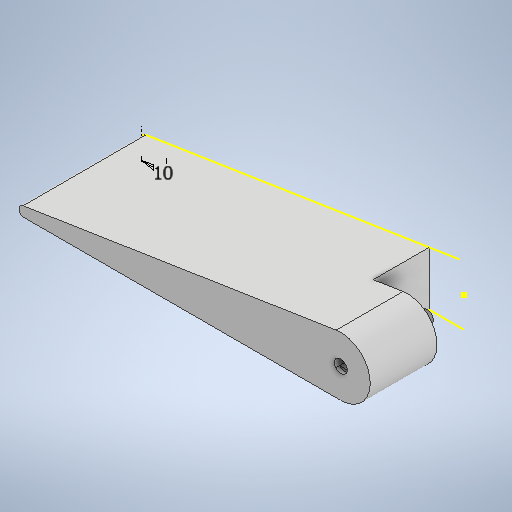
# Autodesk Inventor part: 13042025-02
Saved by Autodesk Inventor 2025.2 (Build 292293000, 293)
## iProperties
Created: 2026-04-13
Part Number: 13042025-02
Material: Generic
Document SubType Name: Modeling
Designer: Oski
Density: 1 g/cm^3
Appearance: Default
Author: Oski
Autodesk Inventor part; units mm, degrees
ref_plane "YZ Plane" through (0, 0, 0) normal (1, 0, 0) x (0, 1, 0)
ref_plane "XZ Plane" through (0, 0, 0) normal (0, 1, 0) x (-1, 0, 0)
ref_plane "XY Plane" through (0, 0, 0) normal (0, 0, 1) x (1, 0, 0)
sketch "Sketch1" plane through (0, 0, 0) normal (0, 0, 1) x (1, 0, 0)
  line L0 (-12, 12) -> (12, 12)
  line L1 (12, 12) -> (12, -12)
  line L2 (12, -12) -> (-12, -12)
  line L3 (-12, -12) -> (-12, 12)
  line L4 (0, 0) -> (0, 12) construction
  line L5 (0, 0) -> (0, -12) construction
  line L6 (0, 0) -> (-12, 0) construction
  dimension "d0" = 24
  dimension "d1" = 24
  constraints: 14 end point, 3 midpoint, 3 perpendicular, 2 equal length, 2 parallel, 1 horizontal, 1 point on line
  measures "d0" distance of L0.start L0.end
  measures "d1" distance of L2.end L0.start
extrude "Extrusion1" add sketch "Sketch1" along normal blind 27.2
fillet "Fillet2" radius 12 4 edges at (12, 12, 13.6) (12, -12, 13.6) (-12, 12, 13.6) (-12, -12, 13.6)
sketch "Sketch2" plane through (0, 0, 27.2) normal (0, 0, 1) x (1, 0, 0)
  line L0 (2.1125, -1.6) -> (-2.1125, -1.6)
  line L1 (2.1125, 1.6) -> (-2.1125, 1.6)
  arc A0 (2.1125, -1.6) -> (2.1125, 1.6) centre (0, 0) ccw
  arc A1 (-2.1125, 1.6) -> (-2.1125, -1.6) centre (0, 0) ccw
  point P0 (2.65, 0)
  point P1 (-2.65, 0)
  dimension "d9" = 2.65
  dimension "d10" = 3.2
  constraints: 6 point on circle, 4 end point, 2 centre point, 2 coincident, 2 horizontal, 1 concentric, 1 parallel
  measures "d9" radius of A0
  measures "d10" distance between parallel lines of L1 L0
extrude "Extrusion2" cut sketch "Sketch2" against normal blind 8
sketch "Sketch3" plane through (0, 0, 27.2) normal (0, 0, 1) x (1, 0, 0)
  circle A0 centre (0, 0) radius 2.6
  dimension "d13" = 5.2
  constraints: 1 centre point, 1 coincident
  measures "d13" diameter of A0
extrude "Extrusion3" cut sketch "Sketch3" against normal blind 1.6
sketch "Sketch4" plane through (0, 0, 0) normal (0, 0, -1) x (-1, 0, 0)
  arc A0 (-2.1125, 1.6) -> (-2.1125, -1.6) centre (0, 0) ccw projected
  circle A1 centre (0, 0) radius 3.25
  dimension "d17" = 6.5
  constraints: 1 centre point, 1 coincident
  measures "d17" diameter of A1
extrude "Extrusion4" add sketch "Sketch4" along normal blind 3
sketch "Sketch5" plane through (0, 0, -3) normal (0, 0, -1) x (-1, 0, 0)
  circle A0 centre (0, 0) radius 2.45
  dimension "d20" = 4.9
  constraints: 1 centre point, 1 coincident
  measures "d20" diameter of A0
extrude "Extrusion5" add sketch "Sketch5" along normal blind 5
sketch "Sketch7" plane through (0, 0, 27.2) normal (0, 0, 1) x (1, 0, 0)
  circle A0 centre (0, 0) radius 12 projected
  line L0 (0, -12) -> (-129, -12)
  line L1 (-129.3082, -8.0239) -> (-1.8494, 11.8566)
  line L2 (12, -13.9286) -> (12, 16.8355)
  circle A1 centre (0, 0) radius 12 projected
  arc A2 (-129.3082, -8.0239) -> (-129, -12) centre (-129, -10) ccw
  line L3 (-131, -17.4392) -> (-131, 0.6536)
  point P0 (-1.8494, 11.8566)
  dimension "d36" = 2
  dimension "d38" = 143
  constraints: 8 end point, 6 tangent, 3 point on circle, 2 vertical, 1 centre point, 1 horizontal, 2 other
  measures "d36" radius of A2
  measures "d38" distance between parallel lines of L2 L3
extrude "Extrusion7" add sketch "Sketch7" against normal blind 27.2 contours A0 L0 A2 L1
sketch "Sketch8" plane through (0, 0, 0) normal (0, 0, -1) x (-1, 0, 0)
  line L0 (0, -12) -> (129, -12) projected
  line L1 (14, -12) -> (14, 9.9614)
  line L2 (129.3082, -8.0239) -> (1.8494, 11.8566) projected
  arc A0 (1.8494, 11.8566) -> (0, -12) centre (0, 0) ccw projected
  line L3 (14, 9.9614) -> (129.3082, -8.0239)
  arc A1 (129, -12) -> (129.3082, -8.0239) centre (129, -10) ccw projected
  line L4 (129, -12) -> (14, -12)
  dimension "d39" = 14
  constraints: 6 end point, 2 point on line, 1 perpendicular, 1 tangent, 1 vertical
  measures "d39" distance from line of A0.centre L1
extrude "Extrusion8" add sketch "Sketch8" along normal blind 22.8 contours L1 L2 A1 L0
sketch "Sketch9" plane through (0, 0, -22.8) normal (0, 0, -1) x (-1, 0, 0)
  arc A0 (129, -12) -> (129.3082, -8.0239) centre (129, -10) ccw projected
  line L0 (131, -5.9887) -> (131, -16.219) construction
  arc A1 (129, -12) -> (129.3082, -8.0239) centre (129, -10) ccw projected
  line L1 (1.8494, 11.8566) -> (129.3082, -8.0239) projected
  line L2 (121, -6.728) -> (121, -12) construction
  line L3 (129, -12) -> (0, -12) projected
  point P0 (0, 0)
  dimension "d43" = 10
  constraints: 4 end point, 2 point on line, 2 vertical, 1 tangent
  measures "d43" distance between parallel lines of L2 L0
body "Solid1"
